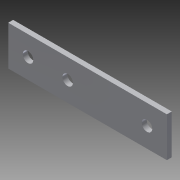
# Autodesk Inventor part: Gusset 3
Saved by Autodesk Inventor 2014 SP1 (Build 180222100, 222)
## iProperties
Created: 2013-01-31
Part Number: Gusset 3
Material: Aluminum 6061
Document SubType Name: Modeling
Designer: actoennies
Density: 2.71 g/cm^3
Mass: 21.279 g
Surface Area: 59.5479 cm^2
Volume: 7.85204 cm^3
Appearance: Aluminum - Flat
Author: actoennies
Autodesk Inventor part; units mm, degrees
ref_plane "YZ Plane" through (0, 0, 0) normal (1, 0, 0) x (0, 1, 0)
ref_plane "XZ Plane" through (0, 0, 0) normal (0, 1, 0) x (-1, 0, 0)
ref_plane "XY Plane" through (0, 0, 0) normal (0, 0, 1) x (1, 0, 0)
sketch "Sketch1" plane through (0, 0, 0) normal (0, 0, 1) x (1, 0, 0)
  line L0 (0, 0) -> (0, 25.4)
  line L1 (0, 25.4) -> (101.6, 25.4)
  line L2 (101.6, 25.4) -> (101.6, 0)
  line L3 (101.6, 0) -> (0, 0)
  circle A0 centre (22.225, 12.7) radius 3.3782
  circle A1 centre (88.9, 12.7) radius 3.3782
  circle A2 centre (53.975, 12.7) radius 3.3782
  dimension "d0" = 25.4
  dimension "d1" = 101.6
  dimension "d2" = 6.7564
  dimension "d3" = 6.7564
  dimension "d4" = 22.225
  dimension "d5" = 12.7
  dimension "d6" = 12.7
  dimension "d7" = 12.7
  dimension "d10" = 6.7564
  dimension "d11" = 31.75
  dimension "d14" = 12.7
  constraints: 8 end point, 3 centre point, 2 parallel, 1 perpendicular, 1 vertical
  measures "d0" distance of L0.start L0.end
  measures "d1" distance of L0.end L1.end
  measures "d2" diameter of A0
  measures "d3" diameter of A1
  measures "d4" distance from line of L0 A0.centre
  measures "d5" distance from line of L3 A0.centre
  measures "d6" distance from line of L2 A1.centre
  measures "d7" distance from line of L3 A1.centre
  measures "d10" diameter of A2
  measures "d11" distance of A2.centre A0.centre
  measures "d14" distance from line of L3 A2.centre
extrude "Extrusion2" add sketch "Sketch1" along normal blind 3.175
body "Solid2"
